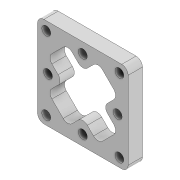
# Autodesk Inventor part: 30_Adapter_AS5600_rotational_enocder_nema12
Saved by Autodesk Inventor 2022 (Build 260153000, 153)
## iProperties
Created: 2023-07-28
Part Number: 30_Adapter_AS5600_rotational_enocder_nema12
Material: Generisch
Document SubType Name: Modeling
Designer: diederichbenedict
Density: 1 g/cm^3
Appearance: Vorgabe
Author: diederichbenedict
Autodesk Inventor part; units mm, degrees
ref_plane "YZ Plane" through (0, 0, 0) normal (1, 0, 0) x (0, 1, 0)
ref_plane "XZ Plane" through (0, 0, 0) normal (0, 1, 0) x (-1, 0, 0)
ref_plane "XY Plane" through (0, 0, 0) normal (0, 0, 1) x (1, 0, 0)
sketch "Skizze5" plane through (0, 0, 0) normal (0, 0, 1) x (1, 0, 0)
  line L0 (-8.1928, -13.75) -> (8.1928, -13.75) projected
  arc A0 (13.75, -8.1928) -> (8.1928, -13.75) centre (11.5, -11.5) ccw projected
  line L1 (13.75, -8.1928) -> (13.75, 8.1928) projected
  arc A1 (8.1928, 13.75) -> (13.75, 8.1928) centre (11.5, 11.5) ccw projected
  line L2 (8.1928, 13.75) -> (-8.1928, 13.75) projected
  arc A2 (-13.75, 8.1928) -> (-8.1928, 13.75) centre (-11.5, 11.5) ccw projected
  line L3 (-13.75, 8.1928) -> (-13.75, -8.1928) projected
  arc A3 (-8.1928, -13.75) -> (-13.75, -8.1928) centre (-11.5, -11.5) ccw projected
  circle A4 centre (0, 0) radius 4 projected
  circle A5 centre (0, 0) radius 2.2643 construction
  circle A6 centre (0, 10.9602) radius 2 construction
  circle A7 centre (0, -10.9602) radius 2 construction
  circle A8 centre (10.9602, 0) radius 2 construction
  circle A9 centre (-10.9602, 0) radius 2 construction
  line L4 (13.0815, -2.8284) -> (2.8284, -13.0815) construction
  arc A10 (13.0815, -2.8284) -> (13.0815, 2.8284) centre (10.253, 0) ccw construction
  line L5 (2.8284, 13.0815) -> (13.0815, 2.8284) construction
  arc A11 (2.8284, 13.0815) -> (-2.8284, 13.0815) centre (0, 10.253) ccw construction
  line L6 (-13.0815, 2.8284) -> (-2.8284, 13.0815) construction
  arc A12 (-13.0815, 2.8284) -> (-13.0815, -2.8284) centre (-10.253, 0) ccw construction
  line L7 (-2.8284, -13.0815) -> (-13.0815, -2.8284) construction
  arc A13 (-2.8284, -13.0815) -> (2.8284, -13.0815) centre (0, -10.253) ccw construction
  arc A14 (14.25, 12.25) -> (12.25, 14.25) centre (12.25, 12.25) ccw construction
  arc A15 (-14.25, -12.25) -> (-12.25, -14.25) centre (-12.25, -12.25) ccw construction
  line L8 (-14.25, -14.25) -> (14.25, -14.25)
  line L9 (14.25, -14.25) -> (14.25, 14.25)
  line L10 (14.25, 14.25) -> (-14.25, 14.25)
  line L11 (-14.25, 14.25) -> (-14.25, -14.25)
  line L12 (-14.25, -14.25) -> (14.25, 14.25) construction
  line L13 (14.25, -14.25) -> (-14.25, 14.25) construction
  circle A16 centre (10.9602, 0) radius 1.4
  circle A17 centre (0, 10.9602) radius 1.4
  circle A18 centre (0, -10.9602) radius 1.4
  circle A19 centre (-10.9602, 0) radius 1.4
  line L14 (-11.1369, 4.773) -> (4.773, -11.1369)
  line L15 (4.773, -11.1369) -> (11.1369, -4.773)
  line L16 (11.1369, -4.773) -> (-4.773, 11.1369)
  line L17 (-4.773, 11.1369) -> (-11.1369, 4.773)
  line L18 (-11.1369, 4.773) -> (11.1369, -4.773) construction
  line L19 (4.773, -11.1369) -> (-4.773, 11.1369) construction
  line L20 (11.1369, 4.773) -> (-4.773, -11.1369)
  line L21 (-4.773, -11.1369) -> (-11.1369, -4.773)
  line L22 (-11.1369, -4.773) -> (4.773, 11.1369)
  line L23 (4.773, 11.1369) -> (11.1369, 4.773)
  line L24 (11.1369, 4.773) -> (-11.1369, -4.773) construction
  line L25 (-4.773, -11.1369) -> (4.773, 11.1369) construction
  circle A20 centre (11.5, 11.5) radius 1.4 projected
  circle A21 centre (11.5, -11.5) radius 1.4 projected
  circle A22 centre (-11.5, -11.5) radius 1.4 projected
  circle A23 centre (-11.5, 11.5) radius 1.4 projected
  point P0 (0, 0)
  point P1 (0, -6.364)
  point P2 (-6.364, 0)
  point P3 (0, 6.364)
  point P4 (6.364, 0)
  dimension "d13" = 2.8
  dimension "d14" = 2.8
  dimension "d15" = 2.8
  dimension "d16" = 2.8
  dimension "d17" = 9
  dimension "d18" = 9
  constraints: 36 end point, 6 midpoint, 6 parallel, 4 centre point, 4 coincident, 3 perpendicular, 1 horizontal
  measures "d13" diameter of A16
  measures "d14" diameter of A17
  measures "d15" diameter of A18
  measures "d16" diameter of A19
  measures "d17" distance of L15.end L14.end
  measures "d18" distance of L20.end L21.end
extrude "Extrusion4" add sketch "Skizze5" along normal blind 4.5 contours A3 L3 A2 L2 A1 L1 A0 L0 | L11 L10 L9 L8
fillet "Rundung2" radius 2 16 edges at (14.25, 14.25, 2.25) (14.25, -14.25, 2.25) (-14.25, -14.25, 2.25) (-14.25, 14.25, 2.25) (0, 6.364, 2.25) (4.773, 11.1369, 2.25) (-4.773, 11.1369, 2.25) (-11.1369, 4.773, 2.25) (-6.364, 0, 2.25) (-11.1369, -4.773, 2.25) (-4.773, -11.1369, 2.25) (0, -6.364, 2.25) (4.773, -11.1369, 2.25) (11.1369, -4.773, 2.25) (6.364, 0, 2.25) (11.1369, 4.773, 2.25)
sketch "Skizze6" plane through (0, 0, 0) normal (0, 0, -1) x (-1, 0, 0)
  line L0 (-14.25, -12.25) -> (-14.25, -8.1928) projected
  arc A0 (-14.25, -8.1928) -> (-13.4687, -8.6062) centre (-13.75, -8.1928) ccw projected
  arc A1 (-8.6062, -13.4688) -> (-13.4687, -8.6062) centre (-11.5, -11.5) ccw projected
  arc A2 (-8.6062, -13.4688) -> (-8.1928, -14.25) centre (-8.1928, -13.75) ccw projected
  line L1 (-8.1928, -14.25) -> (-12.25, -14.25) projected
  arc A3 (-14.25, -12.25) -> (-12.25, -14.25) centre (-12.25, -12.25) ccw projected
  circle A4 centre (-11.5, -11.5) radius 1.4 projected
  line L2 (8.1928, 14.25) -> (12.25, 14.25) projected
  arc A5 (14.25, 12.25) -> (12.25, 14.25) centre (12.25, 12.25) ccw projected
  line L3 (14.25, 12.25) -> (14.25, 8.1928) projected
  arc A6 (14.25, 8.1928) -> (13.4688, 8.6062) centre (13.75, 8.1928) ccw projected
  arc A7 (8.6062, 13.4688) -> (13.4688, 8.6062) centre (11.5, 11.5) ccw projected
  arc A8 (8.6062, 13.4688) -> (8.1928, 14.25) centre (8.1928, 13.75) ccw projected
  circle A9 centre (11.5, 11.5) radius 1.4 projected
  point P0 (0, 0)
extrude "Extrusion5" [suppressed]
